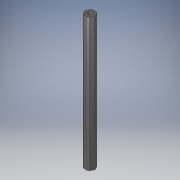
# Autodesk Inventor part: ThunderHex_6.5inch
Saved by Autodesk Inventor 2018 (Build 220112000, 112)
## iProperties
Created: 2017-09-10
Part Number: ThunderHex_6.5inch
Material: Generic
Document SubType Name: Modeling
Designer: snipe
Density: 1 g/cm^3
Appearance: Steel - Polished
Author: snipe
Autodesk Inventor part; units mm, degrees
ref_plane "YZ Plane" through (0, 0, 0) normal (1, 0, 0) x (0, 1, 0)
ref_plane "XZ Plane" through (0, 0, 0) normal (0, 1, 0) x (-1, 0, 0)
ref_plane "XY Plane" through (0, 0, 0) normal (0, 0, 1) x (1, 0, 0)
sketch "Sketch1" plane through (0, 0, 0) normal (0, 1, 0) x (-1, 0, 0)
  line L0 (0, -9.0532) -> (0, 9.0532) projected
  line L1 (-9.625, 0) -> (9.625, 0) projected
  line L2 (-4.287, -5.3747) -> (-6.7981, -1.0253)
  line L3 (-6.7981, 1.0253) -> (-4.287, 5.3747)
  line L4 (-2.5111, 6.4) -> (2.5111, 6.4)
  line L5 (4.287, 5.3747) -> (6.7981, 1.0253)
  line L6 (6.7981, -1.0253) -> (4.287, -5.3747)
  line L7 (2.5111, -6.4) -> (-2.5111, -6.4)
  circle A0 centre (0, 0) radius 2.55
  arc A1 (2.5111, -6.4) -> (4.287, -5.3747) centre (0, 0) ccw
  arc A2 (-4.287, -5.3747) -> (-2.5111, -6.4) centre (0, 0) ccw
  arc A3 (-6.7981, 1.0253) -> (-6.7981, -1.0253) centre (0, 0) ccw
  arc A4 (-2.5111, 6.4) -> (-4.287, 5.3747) centre (0, 0) ccw
  arc A5 (6.7981, -1.0253) -> (6.7981, 1.0253) centre (0, 0) ccw
  arc A6 (4.287, 5.3747) -> (2.5111, 6.4) centre (0, 0) ccw
  dimension "d0" = 12.8
  dimension "d5" = 5.1
  constraints: 12 end point, 12 point on circle, 7 centre point, 3 coincident, 1 horizontal, 7 other
  measures "d0" distance between parallel lines of L4 L7
  measures "d5" diameter of A0
extrude "Extrusion2" add sketch "Sketch1" along normal blind 184.15 contours L7 A2 L2 A3 L1 A0 L0 | L0 A0 L1 A5 L6 A1 L7 | L1 A3 L3 A4 L4 L0 A0 | A0 L0 L4 A6 L5 A5 L1
body "Solid2"
